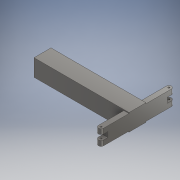
# Autodesk Inventor part: Ciągaczka
Saved by Autodesk Inventor 2017 (Build 210142000, 142)
## iProperties
Created: 2018-05-29
Part Number: Ciągaczka
Material: Stainless Steel, 440C
Document SubType Name: Modeling
Designer: Pies
Density: 7.75 g/cm^3
Appearance: Semi-Polished
Author: Pies
Autodesk Inventor part; units mm, degrees
ref_plane "YZ Plane" through (0, 0, 0) normal (1, 0, 0) x (0, 1, 0)
ref_plane "XZ Plane" through (0, 0, 0) normal (0, 1, 0) x (-1, 0, 0)
ref_plane "XY Plane" through (0, 0, 0) normal (0, 0, 1) x (1, 0, 0)
sketch "Sketch1" plane through (0, 0, 0) normal (0, 0, 1) x (1, 0, 0)
  line L0 (1.5, 0) -> (1.5, 20)
  line L1 (-1.5, 20) -> (-1.5, 1.5)
  line L2 (1.5, 0) -> (1.5, -20)
  line L3 (-1.5, -20) -> (-1.5, -1.5)
  circle A0 centre (0, 20) radius 0.5
  arc A1 (1.5, 20) -> (-1.5, 20) centre (0, 20) ccw
  circle A2 centre (0, -20) radius 0.5
  arc A3 (-1.5, -20) -> (1.5, -20) centre (0, -20) ccw
  line L4 (-1.5, 1.5) -> (-1.5, -1.5)
  point P0 (0, 0)
  constraints: 10 end point, 4 centre point, 4 point on circle, 2 coincident, 2 tangent, 1 vertical
extrude "Extrusion1" add sketch "Sketch1" along normal blind 9
sketch "Sketch3" plane through (-1.5, -20, 0) normal (-1, 0, 0) x (0, 0, 1)
  line L0 (9, 0) -> (9, 40) projected
  line L1 (9, 20) -> (0, 20)
  line L2 (0, 0) -> (0, 40) projected
  line L3 (9.5, 15) -> (-0.5, 15)
  line L4 (-0.5, 15) -> (-0.5, 25)
  line L5 (-0.5, 25) -> (9.5, 25)
  line L6 (9.5, 25) -> (9.5, 15)
  line L7 (9.5, 15) -> (-0.5, 25) construction
  line L8 (-0.5, 15) -> (9.5, 25) construction
  point P0 (4.5, 20)
  dimension "d29" = 10
  dimension "d30" = 10
  constraints: 14 end point, 5 midpoint, 2 parallel, 1 horizontal, 1 perpendicular
  measures "d29" distance of L4.end L5.end
  measures "d30" distance of L3.end L4.end
extrude "Extrusion2" add sketch "Sketch3" along normal blind 53 and the other way blind 3
sketch "Sketch5" plane through (-54.5, -20, 0) normal (-1, 0, 0) x (0, 0, 1)
  line L0 (0, 15) -> (-0.5, 15) construction
  line L1 (9.5, 25) -> (9.5, 15) construction
  line L2 (-0.5, 15) -> (9.5, 25) construction
  point P0 (0, 20)
  point P1 (4.5, 20)
  constraints: 2 end point, 1 midpoint
hole "Hole2" at (-54.5, 0, 4.5) direction (1, 0, 0) diameter 9 depth 16 clearance for "Hex Head Cap Screw ISO 24017" size "M8" standard "ISO"
sketch "Sketch6" plane through (1.5, 20, 9) normal (1, 0, 0) x (0, 0, -1)
  line L0 (9, -20) -> (-0.0817, -20) construction
  line L1 (6, -37.5) -> (6, -41.5)
  line L2 (6, -37.5) -> (3, -37.5)
  line L3 (3, -37.5) -> (3, -41.5)
  line L4 (6, -41.5) -> (3, -41.5)
  line L5 (6, -2.5) -> (6, 1.5)
  line L6 (6, -2.5) -> (3, -2.5)
  line L7 (3, -2.5) -> (3, 1.5)
  line L8 (6, 1.5) -> (3, 1.5)
  constraints: 18 end point, 4 symmetric about line, 2 perpendicular, 1 horizontal
extrude "Extrusion3" cut sketch "Sketch6" against normal through all
body "Solid1"
